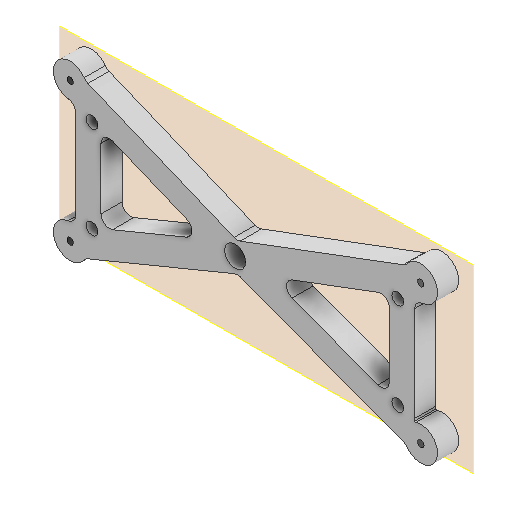
# Autodesk Inventor part: ESP32ParasiteMicroscope_lid_v0
Saved by Autodesk Inventor 2022 (Build 260153000, 153)
## iProperties
Created: 2022-02-02
Part Number: ESP32ParasiteMicroscope_lid_v0
Material: Generisch
Document SubType Name: Modeling
Designer: diederichbenedict
Density: 1 g/cm^3
Appearance: Vorgabe
Author: diederichbenedict
Autodesk Inventor part; units mm, degrees
ref_plane "YZ Plane" through (0, 0, 0) normal (1, 0, 0) x (0, 1, 0)
ref_plane "XZ Plane" through (0, 0, 0) normal (0, 1, 0) x (-1, 0, 0)
ref_plane "XY Plane" through (0, 0, 0) normal (0, 0, 1) x (1, 0, 0)
ref_plane "Arbeitsebene1" through (0, 0, 15) normal (0, 0, 1) x (1, 0, 0)
sketch "Skizze1" plane through (0, 0, 15) normal (0, 0, 1) x (1, 0, 0)
  circle A0 centre (-2.443914, 0) radius 3.45
  circle A1 centre (-41.53745, 16.48745) radius 1.15
  circle A2 centre (41.53745, 16.48745) radius 1.4
  circle A3 centre (41.53745, -16.48745) radius 1.4
  circle A4 centre (-41.53745, -16.48745) radius 1.4
  arc A5 (-41.53745, 19.48745) -> (-44.53745, 16.48745) centre (-41.53745, 16.48745) ccw
  line L0 (-44.53745, 16.48745) -> (-44.53745, -16.48745)
  arc A6 (-44.53745, -16.48745) -> (-41.53745, -19.48745) centre (-41.53745, -16.48745) ccw
  line L1 (-41.53745, -19.48745) -> (41.53745, -19.48745)
  arc A7 (41.53745, -19.48745) -> (44.53745, -16.48745) centre (41.53745, -16.48745) ccw
  line L2 (44.53745, -16.48745) -> (44.53745, 16.48745)
  arc A8 (44.53745, 16.48745) -> (41.53745, 19.48745) centre (41.53745, 16.48745) ccw
  line L3 (41.53745, 19.48745) -> (-41.53745, 19.48745)
  circle A9 centre (41.53745, 16.48745) radius 1.4
  circle A10 centre (41.53745, -16.48745) radius 1.4
  circle A11 centre (-2.443914, 0) radius 3.45
  circle A12 centre (-41.53745, -16.48745) radius 1.4
  circle A13 centre (-41.53745, 16.48745) radius 1.15
  circle A14 centre (-41.53745, 16.48745) radius 3
  circle A15 centre (-41.53745, -16.48745) radius 3
  circle A16 centre (41.53745, 16.48745) radius 3
  circle A17 centre (41.53745, -16.48745) radius 3
  line L4 (-1.966099, 3.416752) -> (-40.393905, 19.26095)
  line L5 (-1.966099, 3.416752) -> (40.48635, 19.297288)
  line L6 (-1.966099, -3.416752) -> (40.48635, -19.297288)
  line L7 (-1.966099, -3.416752) -> (-40.393905, -19.26095)
  line L8 (-9.419799, 0) -> (-42.680994, 13.713949)
  line L9 (-9.419799, 0) -> (-42.680994, -13.713949)
  line L10 (42.588549, 13.677612) -> (6.025041, 0)
  line L11 (6.025041, 0) -> (42.588549, -13.677612)
  circle A18 centre (-41.53745, 16.48745) radius 4
  circle A19 centre (-41.53745, -16.48745) radius 4
  circle A20 centre (41.53745, 16.48745) radius 4
  circle A21 centre (41.53745, -16.48745) radius 4
  circle A22 centre (-2.443914, 0) radius 2.5
  line L12 (-40.234996, 12.705438) -> (-34.234996, 12.705438)
  line L13 (-34.234996, 12.705438) -> (-34.234996, -12.705438)
  line L14 (-34.234996, -12.705438) -> (-40.234996, -12.705438)
  line L15 (-40.234996, -12.705438) -> (-40.234996, 12.705438)
  line L16 (40.110505, 12.750629) -> (34.110505, 12.750629)
  line L17 (34.110505, 12.750629) -> (34.110505, -12.705438)
  line L18 (34.110505, -12.705438) -> (40.110505, -12.705438)
  line L19 (40.110505, -12.705438) -> (40.110505, 12.750629)
  point P0 (0, 0)
  point P1 (-40.234996, 12.705438)
  point P2 (-40.234996, -12.705438)
  point P3 (-37.947908, -18.252439)
  point P4 (38.008306, -18.370305)
  point P5 (40.110505, -12.750629)
  point P6 (40.110505, 12.750629)
  point P7 (38.008306, 18.370305)
  point P8 (-37.947908, 18.252439)
  point P9 (34.110505, 10.50616)
  point P10 (34.110505, -10.50616)
  point P11 (39.989697, -12.705438)
  point P12 (-34.234996, -10.231573)
  point P13 (-34.234996, 10.231573)
  dimension "d2" = 8
  dimension "d4" = 8
  dimension "d0" = 0
  dimension "d1" = 0
  dimension "d3" = 8
  dimension "d5" = 8
  dimension "d6" = 5
  dimension "d22" = 6
  dimension "d23" = 6
  constraints: 32 end point, 11 point on circle, 9 coincident, 8 parallel, 7 centre point, 7 tangent, 3 concentric, 3 point on line, 2 horizontal, 2 perpendicular, 6 other
  measures "d0" vertical distance of L8.start A0.centre
  measures "d1" vertical distance of A0.centre L10.end
  measures "d3" diameter of A19
  measures "d5" diameter of A21
  measures "d6" diameter of A22
  measures "d22" distance of L13.end L14.end
  measures "d23" distance of L18.end L17.end
extrude "Extrusion1" add sketch "Skizze1" along normal blind 5 contours A0 | A0 L5 A20 L16 L17 L10 L11 L18 A21 L6 | A0 L7 A19 L14 L13 L9 L8 L12 A18 L4 | A18 L8 A14 L4 | L4 A14 L3 A18 | A20 L3 A16 L5 | L5 A16 L10 A20 | A21 L11 A17 L6 | L6 A17 L1 A21 | A19 L1 A15 L7 | L7 A15 L9 A19 | A14 A5 | L3 A5 L0 A18 | A16 A8 | A20 L2 A8 L3 | L19 L18 L11 L17 L10 | L10 A16 L2 A20 | L10 L17 L16 | A17 A7 | A21 L2 A17 L11 | L1 A7 L2 A21 | A15 A6 | A19 L0 A6 L1 | A18 L0 A14 L8 | L12 L13 L8 | L8 L13 L9 L15 | L18 L17 L11 | A19 L9 A15 L0 | L9 L13 L14 | A1 | A2 | A3 | A4
sketch "Skizze2" plane through (0, 0, 15) normal (0, 0, -1) x (-1, 0, 0)
  circle A0 centre (41.53745, -16.48745) radius 1.4
  circle A1 centre (41.53745, 16.48745) radius 1.15
  circle A2 centre (-41.53745, 16.48745) radius 1.4
  circle A3 centre (-41.53745, 16.48745) radius 1.4
  circle A4 centre (41.53745, -16.48745) radius 1.4
  circle A5 centre (-41.53745, -16.48745) radius 1.4
  circle A6 centre (41.53745, 16.48745) radius 1.15
  arc A7 (41.53745, -19.48745) -> (44.53745, -16.48745) centre (41.53745, -16.48745) ccw
  line L0 (44.53745, -16.48745) -> (44.53745, 16.48745)
  arc A8 (44.53745, 16.48745) -> (41.53745, 19.48745) centre (41.53745, 16.48745) ccw
  arc A9 (-41.53745, 19.48745) -> (-44.53745, 16.48745) centre (-41.53745, 16.48745) ccw
  line L1 (-44.53745, 16.48745) -> (-44.53745, -16.48745)
  arc A10 (-44.53745, -16.48745) -> (-41.53745, -19.48745) centre (-41.53745, -16.48745) ccw
  line L2 (-41.53745, -19.48745) -> (41.53745, -19.48745)
  line L3 (41.53745, 19.48745) -> (-41.53745, 19.48745)
  line L4 (19.590354, -14.373892) -> (-10.409646, -14.373892)
  line L5 (-10.409646, -14.373892) -> (-10.409646, -8.373892)
  line L6 (-10.409646, -8.373892) -> (19.590354, -8.373892)
  line L7 (19.590354, -8.373892) -> (19.590354, -14.373892)
  line L8 (19.657354, 8.753108) -> (-10.342646, 8.753108)
  line L9 (-10.342646, 8.753108) -> (-10.342646, 14.753108)
  line L10 (-10.342646, 14.753108) -> (19.657354, 14.753108)
  line L11 (19.657354, 14.753108) -> (19.657354, 8.753108)
  point P0 (0, 0)
hole "Bohrung1" at (-41.53745, -16.48745, 15) at (-41.53745, 16.48745, 15) at (41.53745, 16.48745, 15) at (41.53745, -16.48745, 15) direction (0, 0, 1) diameter 4.9 depth 4 tip angle 118
fillet "Rundung1" radius 2 17 edges at (-37.9479, -18.2524, 17.5) (-1.9661, -3.4168, 17.5) (-37.9479, 18.2524, 17.5) (-1.9661, 3.4168, 17.5) (6.025, 0, 17.5) (-9.4198, 0, 17.5) (38.0083, 18.3703, 17.5) (40.1105, -12.7506, 17.5) (38.0083, -18.3703, 17.5) (-34.235, 10.2316, 17.5) (-34.235, -10.2316, 17.5) (-40.235, 12.7054, 17.5) (-40.235, -12.7054, 17.5) (34.1105, 10.5062, 17.5) (34.1105, -10.5062, 17.5) (40.1105, -12.7054, 17.5) (40.1105, 12.7506, 17.5)
sketch "Skizze4" plane through (0, 0, 20) normal (0, 0, 1) x (1, 0, 0)
  arc A0 (39.989697, -12.705438) -> (40.110505, -12.020868) centre (38.110505, -12.020868) ccw
  line L0 (40.110505, -12.020868) -> (40.110505, 10.514878)
  arc A1 (41.919486, 12.505735) -> (40.110505, 10.514878) centre (42.110505, 10.514878) ccw
  arc A2 (41.919486, 12.505735) -> (38.298633, 18.834803) centre (41.53745, 16.48745) ccw
  arc A3 (37.379958, 18.135254) -> (38.298633, 18.834803) centre (36.679225, 20.008479) ccw
  line L1 (37.379958, 18.135254) -> (-1.22979, 3.692189)
  arc A4 (-2.692885, 3.716414) -> (-1.22979, 3.692189) centre (-1.930523, 5.565414) ccw
  line L2 (-2.692885, 3.716414) -> (-37.327685, 17.996715)
  arc A5 (-38.222698, 18.726293) -> (-37.327685, 17.996715) centre (-36.565322, 19.845715) ccw
  arc A6 (-38.222698, 18.726293) -> (-42.002481, 12.514573) centre (-41.53745, 16.48745) ccw
  arc A7 (-40.234996, 10.528135) -> (-42.002481, 12.514573) centre (-42.234996, 10.528135) ccw
  line L3 (-40.234996, 10.528135) -> (-40.234996, -10.528135)
  arc A8 (-42.002481, -12.514573) -> (-40.234996, -10.528135) centre (-42.234996, -10.528135) ccw
  arc A9 (-42.002481, -12.514573) -> (-38.222698, -18.726293) centre (-41.53745, -16.48745) ccw
  arc A10 (-37.327685, -17.996715) -> (-38.222698, -18.726293) centre (-36.565322, -19.845715) ccw
  line L4 (-37.327685, -17.996715) -> (-2.692885, -3.716414)
  arc A11 (-1.22979, -3.692189) -> (-2.692885, -3.716414) centre (-1.930523, -5.565414) ccw
  line L5 (-1.22979, -3.692189) -> (37.379958, -18.135254)
  arc A12 (38.298633, -18.834803) -> (37.379958, -18.135254) centre (36.679225, -20.008479) ccw
  arc A13 (38.298633, -18.834803) -> (40.467034, -12.633334) centre (41.53745, -16.48745) ccw
  arc A14 (39.989697, -12.705438) -> (40.467034, -12.633334) centre (39.931827, -10.706276) ccw
  circle A15 centre (41.53745, 16.48745) radius 0.785721
  circle A16 centre (-41.53745, -16.48745) radius 0.785721
  circle A17 centre (-41.53745, 16.48745) radius 0.785721
  circle A18 centre (41.53745, -16.48745) radius 0.785721
  line L6 (34.110505, 7.622649) -> (34.110505, -7.622649)
  arc A19 (31.409772, -9.495875) -> (34.110505, -7.622649) centre (32.110505, -7.622649) ccw
  line L7 (31.409772, -9.495875) -> (11.032618, -1.873225)
  arc A20 (11.032618, 1.873225) -> (11.032618, -1.873225) centre (11.733351, 0) ccw
  line L8 (11.032618, 1.873225) -> (31.409772, 9.495875)
  arc A21 (34.110505, 7.622649) -> (31.409772, 9.495875) centre (32.110505, 7.622649) ccw
  circle A22 centre (-2.443914, 0) radius 2.5
  line L9 (-34.234996, -7.243621) -> (-34.234996, 7.243621)
  arc A23 (-31.472633, 9.092621) -> (-34.234996, 7.243621) centre (-32.234996, 7.243621) ccw
  line L10 (-31.472633, 9.092621) -> (-13.904282, 1.849001)
  arc A24 (-13.904282, -1.849001) -> (-13.904282, 1.849001) centre (-14.666645, 0) ccw
  line L11 (-13.904282, -1.849001) -> (-31.472633, -9.092621)
  arc A25 (-34.234996, -7.243621) -> (-31.472633, -9.092621) centre (-32.234996, -7.243621) ccw
  circle A26 centre (-41.53745, -16.48745) radius 2.45
  line L12 (41.305808, 15.736651) -> (-41.53745, 15.736651)
  line L13 (-41.53745, 15.736651) -> (-41.53745, -16.48745)
  line L14 (-41.53745, -16.48745) -> (41.305808, -16.48745)
  line L15 (41.305808, -16.48745) -> (41.305808, 15.736651)
  line L16 (36.110505, 10.541347) -> (-36.342146, 10.541347)
  line L17 (-36.342146, 10.541347) -> (-36.342146, -11.292146)
  line L18 (-36.342146, -11.292146) -> (36.110505, -11.292146)
  line L19 (36.110505, -11.292146) -> (36.110505, 10.541347)
  point P0 (0, 0)
  dimension "d24" = 2
  constraints: 16 end point, 4 parallel, 2 perpendicular, 1 horizontal, 5 other
  measures "d24" distance between parallel lines of L19 L6
hole "Bohrung2" at (36.110505, -11.292146, 20) at (36.110505, 10.541347, 20) at (-36.342146, -11.292146, 20) at (-36.342146, 10.541347, 20) direction (0, 0, -1) diameter 2.8 end through all
